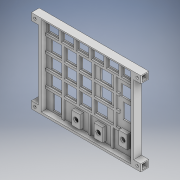
# Autodesk Inventor part: IPC Component Panel
Saved by Autodesk Inventor 2022 (Build 260153000, 153)
## iProperties
Created: 2021-12-31
Part Number: IPC Component Panel
Material: Generic
Document SubType Name: Modeling
Designer: solor
Density: 1 g/cm^3
Appearance: Default
Author: solor
Autodesk Inventor part; units mm, degrees
(part 1 of 2)
ref_plane "YZ Plane" through (0, 0, 0) normal (1, 0, 0) x (0, 1, 0)
ref_plane "XZ Plane" through (0, 0, 0) normal (0, 1, 0) x (-1, 0, 0)
ref_plane "XY Plane" through (0, 0, 0) normal (0, 0, 1) x (1, 0, 0)
sketch "Sketch1" plane through (0, 0, 0) normal (0, 0, 1) x (1, 0, 0)
  line L0 (-9, 0) -> (-9, -9)
  line L1 (-9, -46.5) -> (-9, -59.5)
  line L2 (-9, -97) -> (-9, -106)
  line L3 (-9, -9) -> (0, -9)
  line L4 (0, -9) -> (0, -46.5)
  line L5 (0, -46.5) -> (-9, -46.5)
  line L6 (-9, -59.5) -> (0, -59.5)
  line L7 (0, -59.5) -> (0, -97)
  line L8 (0, -97) -> (-9, -97)
  line L9 (-9, 0) -> (129.8502, 0)
  line L10 (129.8502, -9) -> (120.8502, -9)
  line L11 (120.8502, -9) -> (120.8502, -46.5)
  line L12 (120.8502, -46.5) -> (129.8502, -46.5)
  line L13 (129.8502, -46.5) -> (129.8502, -59.5)
  line L14 (129.8502, -59.5) -> (120.8502, -59.5)
  line L15 (120.8502, -59.5) -> (120.8502, -97)
  line L16 (120.8502, -97) -> (129.8502, -97)
  line L17 (129.8502, -97) -> (129.8502, -106)
  line L18 (-9, -106) -> (129.8502, -106)
  line L19 (129.8502, 0) -> (129.8502, -9)
  circle A0 centre (104.8902, -84.37) radius 6.22
  circle A1 centre (73.6502, -92.18) radius 3.05
  circle A2 centre (45.1902, -92.18) radius 3.05
  line L20 (21.7302, -100.81) -> (21.7302, -81.47)
  line L21 (21.7302, -81.47) -> (11.8502, -81.47)
  line L22 (11.8502, -81.47) -> (11.8502, -100.81)
  line L23 (11.8502, -100.81) -> (21.7302, -100.81)
  line L24 (100.7, -46.82) -> (110.58, -46.82)
  line L25 (110.58, -46.82) -> (110.58, -66.16)
  line L26 (110.58, -66.16) -> (100.7, -66.16)
  line L27 (100.7, -66.16) -> (100.7, -46.82)
  line L28 (5.7515, -17.0785) -> (19.8485, -17.0785)
  line L29 (19.8485, -17.0785) -> (19.8485, -2.9815)
  line L30 (19.8485, -2.9815) -> (5.7515, -2.9815)
  line L31 (5.7515, -2.9815) -> (5.7515, -17.0785)
  line L32 (5.7515, -17.0785) -> (19.8485, -2.9815) construction
  line L33 (19.8485, -17.0785) -> (5.7515, -2.9815) construction
  line L34 (24.8015, -17.0785) -> (38.8985, -17.0785)
  line L35 (38.8985, -17.0785) -> (38.8985, -2.9815)
  line L36 (38.8985, -2.9815) -> (24.8015, -2.9815)
  line L37 (24.8015, -2.9815) -> (24.8015, -17.0785)
  line L38 (24.8015, -17.0785) -> (38.8985, -2.9815) construction
  line L39 (38.8985, -17.0785) -> (24.8015, -2.9815) construction
  line L40 (43.8515, -17.0785) -> (57.9485, -17.0785)
  line L41 (57.9485, -17.0785) -> (57.9485, -2.9815)
  line L42 (57.9485, -2.9815) -> (43.8515, -2.9815)
  line L43 (43.8515, -2.9815) -> (43.8515, -17.0785)
  line L44 (43.8515, -17.0785) -> (57.9485, -2.9815) construction
  line L45 (57.9485, -17.0785) -> (43.8515, -2.9815) construction
  line L46 (62.9015, -17.0785) -> (76.9985, -17.0785)
  line L47 (76.9985, -17.0785) -> (76.9985, -2.9815)
  line L48 (76.9985, -2.9815) -> (62.9015, -2.9815)
  line L49 (62.9015, -2.9815) -> (62.9015, -17.0785)
  line L50 (62.9015, -17.0785) -> (76.9985, -2.9815) construction
  line L51 (76.9985, -17.0785) -> (62.9015, -2.9815) construction
  line L52 (81.9515, -17.0785) -> (96.0485, -17.0785)
  line L53 (96.0485, -17.0785) -> (96.0485, -2.9815)
  line L54 (96.0485, -2.9815) -> (81.9515, -2.9815)
  line L55 (81.9515, -2.9815) -> (81.9515, -17.0785)
  line L56 (81.9515, -17.0785) -> (96.0485, -2.9815) construction
  line L57 (96.0485, -17.0785) -> (81.9515, -2.9815) construction
  line L58 (101.0015, -17.0785) -> (115.0985, -17.0785)
  line L59 (115.0985, -17.0785) -> (115.0985, -2.9815)
  line L60 (115.0985, -2.9815) -> (101.0015, -2.9815)
  line L61 (101.0015, -2.9815) -> (101.0015, -17.0785)
  line L62 (101.0015, -17.0785) -> (115.0985, -2.9815) construction
  line L63 (115.0985, -17.0785) -> (101.0015, -2.9815) construction
  line L64 (9.4915, -37.4985) -> (23.5885, -37.4985)
  line L65 (23.5885, -37.4985) -> (23.5885, -23.4015)
  line L66 (23.5885, -23.4015) -> (9.4915, -23.4015)
  line L67 (9.4915, -23.4015) -> (9.4915, -37.4985)
  line L68 (9.4915, -37.4985) -> (23.5885, -23.4015) construction
  line L69 (23.5885, -37.4985) -> (9.4915, -23.4015) construction
  line L70 (28.5115, -37.4985) -> (42.6085, -37.4985)
  line L71 (42.6085, -37.4985) -> (42.6085, -23.4015)
  line L72 (42.6085, -23.4015) -> (28.5115, -23.4015)
  line L73 (28.5115, -23.4015) -> (28.5115, -37.4985)
  line L74 (28.5115, -37.4985) -> (42.6085, -23.4015) construction
  line L75 (42.6085, -37.4985) -> (28.5115, -23.4015) construction
  line L76 (47.5365, -37.4985) -> (61.6335, -37.4985)
  line L77 (61.6335, -37.4985) -> (61.6335, -23.4015)
  line L78 (61.6335, -23.4015) -> (47.5365, -23.4015)
  line L79 (47.5365, -23.4015) -> (47.5365, -37.4985)
  line L80 (47.5365, -37.4985) -> (61.6335, -23.4015) construction
  line L81 (61.6335, -37.4985) -> (47.5365, -23.4015) construction
  line L82 (72.1215, -37.4985) -> (86.2185, -37.4985)
  line L83 (86.2185, -37.4985) -> (86.2185, -23.4015)
  line L84 (86.2185, -23.4015) -> (72.1215, -23.4015)
  line L85 (72.1215, -23.4015) -> (72.1215, -37.4985)
  line L86 (72.1215, -37.4985) -> (86.2185, -23.4015) construction
  line L87 (86.2185, -37.4985) -> (72.1215, -23.4015) construction
  line L88 (98.5915, -41.7085) -> (112.6885, -41.7085)
  line L89 (112.6885, -41.7085) -> (112.6885, -27.6115)
  line L90 (112.6885, -27.6115) -> (98.5915, -27.6115)
  line L91 (98.5915, -27.6115) -> (98.5915, -41.7085)
  line L92 (98.5915, -41.7085) -> (112.6885, -27.6115) construction
  line L93 (112.6885, -41.7085) -> (98.5915, -27.6115) construction
  line L94 (9.4915, -56.5185) -> (23.5885, -56.5185)
  line L95 (23.5885, -56.5185) -> (23.5885, -42.4215)
  line L96 (23.5885, -42.4215) -> (9.4915, -42.4215)
  line L97 (9.4915, -42.4215) -> (9.4915, -56.5185)
  line L98 (9.4915, -56.5185) -> (23.5885, -42.4215) construction
  line L99 (23.5885, -56.5185) -> (9.4915, -42.4215) construction
  line L100 (28.5065, -56.5185) -> (42.6135, -56.5185)
  line L101 (42.6135, -56.5185) -> (42.6135, -42.4215)
  line L102 (42.6135, -42.4215) -> (28.5065, -42.4215)
  line L103 (28.5065, -42.4215) -> (28.5065, -56.5185)
  line L104 (28.5065, -56.5185) -> (42.6135, -42.4215) construction
  line L105 (42.6135, -56.5185) -> (28.5065, -42.4215) construction
  line L106 (47.5365, -56.5185) -> (61.6335, -56.5185)
  line L107 (61.6335, -56.5185) -> (61.6335, -42.4215)
  line L108 (61.6335, -42.4215) -> (47.5365, -42.4215)
  line L109 (47.5365, -42.4215) -> (47.5365, -56.5185)
  line L110 (47.5365, -56.5185) -> (61.6335, -42.4215) construction
  line L111 (61.6335, -56.5185) -> (47.5365, -42.4215) construction
  line L112 (72.1215, -56.5185) -> (86.2185, -56.5185)
  line L113 (86.2185, -56.5185) -> (86.2185, -42.4215)
  line L114 (86.2185, -42.4215) -> (72.1215, -42.4215)
  line L115 (72.1215, -42.4215) -> (72.1215, -56.5185)
  line L116 (72.1215, -56.5185) -> (86.2185, -42.4215) construction
  line L117 (86.2185, -56.5185) -> (72.1215, -42.4215) construction
  line L118 (9.5, -75.5385) -> (23.58, -75.5385)
  line L119 (23.58, -75.5385) -> (23.58, -61.4415)
  line L120 (23.58, -61.4415) -> (9.5, -61.4415)
  line L121 (9.5, -61.4415) -> (9.5, -75.5385)
  line L122 (9.5, -75.5385) -> (23.58, -61.4415) construction
  line L123 (23.58, -75.5385) -> (9.5, -61.4415) construction
  line L124 (28.5065, -75.5385) -> (42.6135, -75.5385)
  line L125 (42.6135, -75.5385) -> (42.6135, -61.4415)
  line L126 (42.6135, -61.4415) -> (28.5065, -61.4415)
  line L127 (28.5065, -61.4415) -> (28.5065, -75.5385)
  line L128 (28.5065, -75.5385) -> (42.6135, -61.4415) construction
  line L129 (42.6135, -75.5385) -> (28.5065, -61.4415) construction
  line L130 (47.5365, -75.5385) -> (61.6335, -75.5385)
  line L131 (61.6335, -75.5385) -> (61.6335, -61.4415)
  line L132 (61.6335, -61.4415) -> (47.5365, -61.4415)
  line L133 (47.5365, -61.4415) -> (47.5365, -75.5385)
  line L134 (47.5365, -75.5385) -> (61.6335, -61.4415) construction
  line L135 (61.6335, -75.5385) -> (47.5365, -61.4415) construction
  line L136 (66.6017, -75.5385) -> (80.6987, -75.5385)
  line L137 (80.6987, -75.5385) -> (80.6987, -61.4415)
  line L138 (80.6987, -61.4415) -> (66.6017, -61.4415)
  line L139 (66.6017, -61.4415) -> (66.6017, -75.5385)
  line L140 (66.6017, -75.5385) -> (80.6987, -61.4415) construction
  line L141 (80.6987, -75.5385) -> (66.6017, -61.4415) construction
  point P0 (0, 0)
  point P1 (0, 0)
  point P2 (12.8, -10.03)
  point P3 (31.85, -10.03)
  point P4 (50.9, -10.03)
  point P5 (69.95, -10.03)
  point P6 (89, -10.03)
  point P7 (10, -23.88)
  point P8 (16.54, -30.45)
  point P9 (35.56, -30.45)
  point P10 (54.585, -30.45)
  point P11 (79.17, -30.45)
  point P12 (79.17, -49.47)
  point P13 (54.585, -49.47)
  point P14 (35.56, -49.47)
  point P15 (16.54, -49.47)
  point P16 (16.54, -68.49)
  point P17 (35.56, -68.49)
  point P18 (54.585, -68.49)
  point P19 (73.6502, -68.49)
  point P20 (16.7902, -81.47)
  point P21 (21.7302, -91.14)
  point P22 (16.7902, -91.14)
  point P23 (110.58, -56.49)
  point P24 (105.64, -46.82)
  point P25 (105.64, -56.49)
  point P26 (108.05, -10.03)
  point P27 (105.64, -34.66)
  dimension "d56" = 14.097
  dimension "d57" = 14.097
  dimension "d58" = 14.097
  dimension "d59" = 14.097
  dimension "d60" = 14.097
  dimension "d61" = 14.097
  dimension "d62" = 14.097
  dimension "d63" = 14.097
  dimension "d65" = 14.097
  dimension "d66" = 14.097
  dimension "d67" = 14.097
  dimension "d68" = 14.097
  dimension "d69" = 14.097
  dimension "d72" = 14.097
  dimension "d73" = 14.097
  dimension "d74" = 14.097
  dimension "d75" = 14.097
  dimension "d76" = 14.097
  dimension "d77" = 14.097
  dimension "d78" = 14.107
  dimension "d79" = 14.097
  dimension "d80" = 14.097
  dimension "d81" = 14.097
  dimension "d82" = 14.097
  dimension "d83" = 14.097
  dimension "d84" = 14.097
  dimension "d85" = 14.097
  dimension "d86" = 14.097
  dimension "d87" = 14.097
  dimension "d88" = 14.097
  dimension "d89" = 14.107
  dimension "d90" = 14.097
  dimension "d91" = 14.08
  dimension "d92" = 19.34
  dimension "d144" = 6.1
  dimension "d145" = 6.1
  constraints: 284 end point, 42 midpoint, 38 parallel, 33 perpendicular, 27 point on line, 24 horizontal, 5 coincident, 4 vertical, 3 centre point
  measures "d56" distance of L30.end L29.end
  measures "d57" distance of L29.end L28.end
  measures "d58" distance of L36.end L35.end
  measures "d59" distance of L42.end L41.end
  measures "d60" distance of L48.end L47.end
  measures "d61" distance of L54.end L53.end
  measures "d62" distance of L60.end L59.end
  measures "d63" distance of L66.end L65.end
  measures "d65" distance of L72.end L71.end
  measures "d66" distance of L78.end L77.end
  measures "d67" distance of L84.end L83.end
  measures "d68" distance of L90.end L89.end
  measures "d69" distance of L89.end L88.end
  measures "d72" distance of L64.end L65.end
  measures "d73" distance of L70.end L71.end
  measures "d74" distance of L76.end L77.end
  measures "d75" distance of L82.end L83.end
  measures "d76" distance of L94.end L95.end
  measures "d77" distance of L95.end L96.end
  measures "d78" distance of L101.end L102.end
  measures "d79" distance of L100.end L101.end
  measures "d80" distance of L107.end L108.end
  measures "d81" distance of L106.end L107.end
  measures "d82" distance of L113.end L114.end
  measures "d83" distance of L112.end L113.end
  measures "d84" distance of L136.end L137.end
  measures "d85" distance of L137.end L138.end
  measures "d86" distance of L130.end L131.end
  measures "d87" distance of L131.end L132.end
  measures "d88" distance of L124.end L125.end
  measures "d89" distance of L125.end L126.end
  measures "d90" distance of L118.end L119.end
  measures "d91" distance of L119.end L120.end
  measures "d92" distance of L20.start L20.end
  measures "d144" diameter of A1
  measures "d145" diameter of A2
extrude "Extrusion1" add sketch "Sketch1" along normal blind 1.651
sketch "Sketch2" plane through (0, 0, 1.651) normal (0, 0, 1) x (1, 0, 0)
  line L0 (-9, 0) -> (-9, -9) projected
  line L1 (-9, -9) -> (0, -9) projected
  line L2 (0, -9) -> (0, -46.5) projected
  line L3 (0, -46.5) -> (-9, -46.5) projected
  line L4 (-9, -46.5) -> (-9, -59.5) projected
  line L5 (-9, -59.5) -> (0, -59.5) projected
  line L6 (0, -59.5) -> (0, -97) projected
  line L7 (0, -97) -> (-9, -97) projected
  line L8 (-9, -97) -> (-9, -106) projected
  line L9 (-9, -106) -> (129.8502, -106) projected
  line L10 (129.8502, -106) -> (129.8502, -97) projected
  line L11 (129.8502, -97) -> (120.8502, -97) projected
  line L12 (120.8502, -97) -> (120.8502, -59.5) projected
  line L13 (120.8502, -59.5) -> (129.8502, -59.5) projected
  line L14 (129.8502, -59.5) -> (129.8502, -46.5) projected
  line L15 (129.8502, -46.5) -> (120.8502, -46.5) projected
  line L16 (120.8502, -46.5) -> (120.8502, -9) projected
  line L17 (120.8502, -9) -> (129.8502, -9) projected
  line L18 (129.8502, -9) -> (129.8502, 0) projected
  line L19 (129.8502, 0) -> (-9, 0) projected
  circle A0 centre (104.8902, -84.37) radius 6.22 projected
  circle A1 centre (73.6502, -92.18) radius 3.05 projected
  circle A2 centre (45.1902, -92.18) radius 3.05 projected
  line L20 (66.6017, -75.5385) -> (66.6017, -61.4415) projected
  line L21 (66.6017, -61.4415) -> (80.6987, -61.4415) projected
  line L22 (80.6987, -61.4415) -> (80.6987, -75.5385) projected
  line L23 (80.6987, -75.5385) -> (66.6017, -75.5385) projected
  line L24 (47.5365, -75.5385) -> (47.5365, -61.4415) projected
  line L25 (47.5365, -61.4415) -> (61.6335, -61.4415) projected
  line L26 (61.6335, -61.4415) -> (61.6335, -75.5385) projected
  line L27 (61.6335, -75.5385) -> (47.5365, -75.5385) projected
  line L28 (28.5065, -75.5385) -> (28.5065, -61.4415) projected
  line L29 (28.5065, -61.4415) -> (42.6135, -61.4415) projected
  line L30 (42.6135, -61.4415) -> (42.6135, -75.5385) projected
  line L31 (42.6135, -75.5385) -> (28.5065, -75.5385) projected
  line L32 (9.5, -75.5385) -> (9.5, -61.4415) projected
  line L33 (9.5, -61.4415) -> (23.58, -61.4415) projected
  line L34 (23.58, -61.4415) -> (23.58, -75.5385) projected
  line L35 (23.58, -75.5385) -> (9.5, -75.5385) projected
  line L36 (72.1215, -56.5185) -> (72.1215, -42.4215) projected
  line L37 (72.1215, -42.4215) -> (86.2185, -42.4215) projected
  line L38 (86.2185, -42.4215) -> (86.2185, -56.5185) projected
  line L39 (86.2185, -56.5185) -> (72.1215, -56.5185) projected
  line L40 (47.5365, -56.5185) -> (47.5365, -42.4215) projected
  line L41 (47.5365, -42.4215) -> (61.6335, -42.4215) projected
  line L42 (61.6335, -42.4215) -> (61.6335, -56.5185) projected
  line L43 (61.6335, -56.5185) -> (47.5365, -56.5185) projected
  line L44 (28.5065, -56.5185) -> (28.5065, -42.4215) projected
  line L45 (28.5065, -42.4215) -> (42.6135, -42.4215) projected
  line L46 (42.6135, -42.4215) -> (42.6135, -56.5185) projected
  line L47 (42.6135, -56.5185) -> (28.5065, -56.5185) projected
  line L48 (9.4915, -56.5185) -> (9.4915, -42.4215) projected
  line L49 (9.4915, -42.4215) -> (23.5885, -42.4215) projected
  line L50 (23.5885, -42.4215) -> (23.5885, -56.5185) projected
  line L51 (23.5885, -56.5185) -> (9.4915, -56.5185) projected
  line L52 (98.5915, -41.7085) -> (98.5915, -27.6115) projected
  line L53 (98.5915, -27.6115) -> (112.6885, -27.6115) projected
  line L54 (112.6885, -27.6115) -> (112.6885, -41.7085) projected
  line L55 (112.6885, -41.7085) -> (98.5915, -41.7085) projected
  line L56 (72.1215, -37.4985) -> (72.1215, -23.4015) projected
  line L57 (72.1215, -23.4015) -> (86.2185, -23.4015) projected
  line L58 (86.2185, -23.4015) -> (86.2185, -37.4985) projected
  line L59 (86.2185, -37.4985) -> (72.1215, -37.4985) projected
  line L60 (47.5365, -37.4985) -> (47.5365, -23.4015) projected
  line L61 (47.5365, -23.4015) -> (61.6335, -23.4015) projected
  line L62 (61.6335, -23.4015) -> (61.6335, -37.4985) projected
  line L63 (61.6335, -37.4985) -> (47.5365, -37.4985) projected
  line L64 (28.5115, -37.4985) -> (28.5115, -23.4015) projected
  line L65 (28.5115, -23.4015) -> (42.6085, -23.4015) projected
  line L66 (42.6085, -23.4015) -> (42.6085, -37.4985) projected
  line L67 (42.6085, -37.4985) -> (28.5115, -37.4985) projected
  line L68 (9.4915, -37.4985) -> (9.4915, -23.4015) projected
  line L69 (9.4915, -23.4015) -> (23.5885, -23.4015) projected
  line L70 (23.5885, -23.4015) -> (23.5885, -37.4985) projected
  line L71 (23.5885, -37.4985) -> (9.4915, -37.4985) projected
  line L72 (101.0015, -17.0785) -> (101.0015, -2.9815) projected
  line L73 (101.0015, -2.9815) -> (115.0985, -2.9815) projected
  line L74 (115.0985, -2.9815) -> (115.0985, -17.0785) projected
  line L75 (115.0985, -17.0785) -> (101.0015, -17.0785) projected
  line L76 (81.9515, -17.0785) -> (81.9515, -2.9815) projected
  line L77 (81.9515, -2.9815) -> (96.0485, -2.9815) projected
  line L78 (96.0485, -2.9815) -> (96.0485, -17.0785) projected
  line L79 (96.0485, -17.0785) -> (81.9515, -17.0785) projected
  line L80 (62.9015, -17.0785) -> (62.9015, -2.9815) projected
  line L81 (62.9015, -2.9815) -> (76.9985, -2.9815) projected
  line L82 (76.9985, -2.9815) -> (76.9985, -17.0785) projected
  line L83 (76.9985, -17.0785) -> (62.9015, -17.0785) projected
  line L84 (43.8515, -17.0785) -> (43.8515, -2.9815) projected
  line L85 (43.8515, -2.9815) -> (57.9485, -2.9815) projected
  line L86 (57.9485, -2.9815) -> (57.9485, -17.0785) projected
  line L87 (57.9485, -17.0785) -> (43.8515, -17.0785) projected
  line L88 (24.8015, -17.0785) -> (24.8015, -2.9815) projected
  line L89 (24.8015, -2.9815) -> (38.8985, -2.9815) projected
  line L90 (38.8985, -2.9815) -> (38.8985, -17.0785) projected
  line L91 (38.8985, -17.0785) -> (24.8015, -17.0785) projected
  line L92 (5.7515, -17.0785) -> (5.7515, -2.9815) projected
  line L93 (5.7515, -2.9815) -> (19.8485, -2.9815) projected
  line L94 (19.8485, -2.9815) -> (19.8485, -17.0785) projected
  line L95 (19.8485, -17.0785) -> (5.7515, -17.0785) projected
  line L96 (100.7, -46.82) -> (110.58, -46.82) projected
  line L97 (110.58, -46.82) -> (110.58, -66.16) projected
  line L98 (110.58, -66.16) -> (100.7, -66.16) projected
  line L99 (100.7, -66.16) -> (100.7, -46.82) projected
  line L100 (21.7302, -100.81) -> (11.8502, -100.81) projected
  line L101 (11.8502, -100.81) -> (11.8502, -81.47) projected
  line L102 (11.8502, -81.47) -> (21.7302, -81.47) projected
  line L103 (21.7302, -81.47) -> (21.7302, -100.81) projected
  line L104 (19.8485, -2.9815) -> (19.8485, -17.0785) construction
  line L105 (24.8015, -17.0785) -> (24.8015, -2.9815) construction
  line L106 (19.8485, -17.0785) -> (5.7515, -17.0785) construction
  line L107 (61.6335, -23.4015) -> (61.6335, -37.4985) construction
  line L108 (61.6335, -26.759) -> (72.1215, -26.759) construction
  line L109 (72.1215, -37.4985) -> (72.1215, -23.4015) construction
  line L110 (61.6335, -37.4985) -> (47.5365, -37.4985) construction
  line L111 (47.5365, -42.4215) -> (61.6335, -42.4215) construction
  line L112 (9.5, -61.4415) -> (23.58, -61.4415) construction
  line L113 (61.6335, -61.4415) -> (61.6335, -75.5385) construction
  line L114 (61.6335, -68.49) -> (66.6017, -68.49) construction
  line L115 (97.4975, -57.48) -> (97.4975, -60.48)
  line L116 (9.5, -57.48) -> (9.5, -60.48)
  line L117 (97.4975, -38.46) -> (97.4975, -41.46)
  line L118 (9.5, -38.46) -> (9.5, -41.46)
  line L119 (97.4975, -57.48) -> (97.4975, -60.48)
  line L120 (9.5, -57.48) -> (9.5, -60.48)
  line L121 (97.4975, -38.46) -> (97.4975, -41.46)
  line L122 (9.5, -38.46) -> (9.5, -41.46)
  line L123 (97.4975, -76.75) -> (97.4975, -79.75)
  line L124 (9.5, -76.75) -> (9.5, -79.75)
  line L125 (9.5, -38.46) -> (9.5, -41.46)
  line L126 (9.5, -38.46) -> (9.5, -41.46)
  line L127 (7.0425, -18.74) -> (7.0425, -21.74)
  line L128 (7.0425, -18.74) -> (7.0425, -21.74)
  line L129 (113.8947, -18.74) -> (113.8947, -21.74)
  line L130 (22.325, -2.9815) -> (23.825, -2.9815)
  line L131 (23.825, -2.9815) -> (23.825, -18.74)
  line L132 (22.325, -2.9815) -> (20.825, -2.9815)
  line L133 (20.825, -2.9815) -> (20.825, -18.74)
  line L134 (7.0425, -18.74) -> (20.825, -18.74)
  line L135 (23.5885, -23.4015) -> (23.5885, -37.4985) projected
  line L136 (27.55, -21.74) -> (27.55, -38.46)
  line L137 (24.55, -21.74) -> (24.55, -38.46)
  line L138 (9.5, -38.46) -> (24.55, -38.46)
  line L139 (24.55, -21.74) -> (7.0425, -21.74)
  line L140 (9.5, -38.46) -> (24.55, -38.46)
  line L141 (24.55, -100.81) -> (27.55, -100.81)
  line L142 (9.5, -41.46) -> (24.55, -41.46)
  line L143 (9.5, -57.48) -> (24.55, -57.48)
  line L144 (9.5, -57.48) -> (24.55, -57.48)
  line L145 (9.5, -60.48) -> (24.55, -60.48)
  line L146 (24.55, -41.46) -> (24.55, -57.48)
  line L147 (27.55, -57.48) -> (27.55, -41.46)
  line L148 (9.5, -60.48) -> (24.55, -60.48)
  line L149 (9.5, -41.46) -> (24.55, -41.46)
  line L150 (9.5, -76.75) -> (24.55, -76.75)
  line L151 (27.55, -100.81) -> (27.55, -79.75)
  line L152 (27.55, -76.75) -> (27.55, -60.48)
  line L153 (9.5, -79.75) -> (24.55, -79.75)
  line L154 (24.55, -60.48) -> (24.55, -76.75)
  line L155 (24.55, -79.75) -> (24.55, -100.81)
  line L156 (43.8515, -2.9815) -> (57.9485, -2.9815) projected
  line L157 (39.875, -2.9815) -> (39.875, -18.74)
  line L158 (42.875, -18.74) -> (42.875, -2.9815)
  line L159 (23.825, -18.74) -> (39.875, -18.74)
  line L160 (57.9485, -2.9815) -> (57.9485, -17.0785) projected
  line L161 (39.875, -2.9815) -> (42.875, -2.9815)
  line L162 (39.875, -2.9815) -> (39.875, -18.74)
  line L163 (42.875, -18.74) -> (42.875, -2.9815)
  line L164 (39.875, -2.9815) -> (42.875, -2.9815)
  line L165 (58.925, -2.9815) -> (58.925, -18.74)
  line L166 (61.925, -18.74) -> (61.925, -2.9815)
  line L167 (58.925, -2.9815) -> (61.925, -2.9815)
  line L168 (77.975, -2.9815) -> (77.975, -18.74)
  line L169 (80.975, -18.74) -> (80.975, -2.9815)
  line L170 (77.975, -2.9815) -> (80.975, -2.9815)
  line L171 (97.025, -2.9815) -> (97.025, -18.74)
  line L172 (100.025, -18.74) -> (100.025, -2.9815)
  line L173 (97.025, -2.9815) -> (100.025, -2.9815)
  line L174 (42.875, -18.74) -> (58.925, -18.74)
  line L175 (61.925, -18.74) -> (77.975, -18.74)
  line L176 (80.975, -18.74) -> (97.025, -18.74)
  line L177 (100.025, -18.74) -> (113.8947, -18.74)
  line L178 (42.6085, -23.4015) -> (42.6085, -37.4985) projected
  line L179 (47.5365, -37.4985) -> (47.5365, -23.4015) projected
  line L180 (27.55, -38.46) -> (43.5725, -38.46)
  line L181 (27.55, -38.46) -> (43.5725, -38.46)
  line L182 (43.5725, -38.46) -> (43.5725, -21.74)
  line L183 (43.5725, -38.46) -> (43.5725, -21.74)
  line L184 (27.55, -41.46) -> (43.5725, -41.46)
  line L185 (27.55, -41.46) -> (43.5725, -41.46)
  line L186 (46.5725, -21.74) -> (46.5725, -38.46)
  line L187 (46.5725, -21.74) -> (46.5725, -38.46)
  line L188 (43.5725, -21.74) -> (27.55, -21.74)
  line L189 (62.5975, -21.74) -> (46.5725, -21.74)
  line L190 (46.5725, -38.46) -> (62.5975, -38.46)
  line L191 (46.5725, -38.46) -> (62.5975, -38.46)
  line L192 (62.5975, -38.46) -> (62.5975, -21.74)
  line L193 (46.5725, -41.46) -> (62.5975, -41.46)
  line L194 (46.5725, -41.46) -> (62.5975, -41.46)
  line L195 (65.5975, -21.74) -> (65.5975, -38.46)
  line L196 (62.5975, -76.75) -> (62.5975, -60.48)
  line L197 (62.5975, -57.48) -> (62.5975, -41.46)
  line L198 (65.5975, -41.46) -> (65.5975, -57.48)
  line L199 (65.5975, -60.48) -> (65.5975, -76.75)
  line L200 (27.55, -60.48) -> (43.5725, -60.48)
  line L201 (46.5725, -60.48) -> (62.5975, -60.48)
  line L202 (27.55, -60.48) -> (43.5725, -60.48)
  line L203 (46.5725, -60.48) -> (62.5975, -60.48)
  line L204 (43.5725, -76.75) -> (43.5725, -60.48)
  line L205 (43.5725, -57.48) -> (43.5725, -41.46)
  line L206 (43.5725, -76.75) -> (43.5725, -60.48)
  line L207 (43.5725, -57.48) -> (43.5725, -41.46)
  line L208 (27.55, -57.48) -> (43.5725, -57.48)
  line L209 (46.5725, -57.48) -> (62.5975, -57.48)
  line L210 (27.55, -57.48) -> (43.5725, -57.48)
  line L211 (46.5725, -57.48) -> (62.5975, -57.48)
  line L212 (46.5725, -41.46) -> (46.5725, -57.48)
  line L213 (46.5725, -60.48) -> (46.5725, -76.75)
  line L214 (46.5725, -41.46) -> (46.5725, -57.48)
  line L215 (46.5725, -60.48) -> (46.5725, -76.75)
  line L216 (27.55, -76.75) -> (43.5725, -76.75)
  line L217 (46.5725, -76.75) -> (62.5975, -76.75)
  line L218 (65.5975, -76.75) -> (90.6137, -76.75)
  line L219 (93.6137, -76.75) -> (97.4975, -76.75)
  line L220 (65.5975, -60.48) -> (90.6137, -60.48)
  line L221 (93.6137, -60.48) -> (97.4975, -60.48)
  line L222 (65.5975, -60.48) -> (90.6137, -60.48)
  line L223 (93.6137, -60.48) -> (97.4975, -60.48)
  line L224 (93.6137, -60.48) -> (93.6137, -76.75)
  line L225 (90.6137, -76.75) -> (90.6137, -60.48)
  line L226 (65.5975, -57.48) -> (90.6137, -57.48)
  line L227 (93.6137, -57.48) -> (97.4975, -57.48)
  line L228 (65.5975, -57.48) -> (90.6137, -57.48)
  line L229 (93.6137, -57.48) -> (97.4975, -57.48)
  line L230 (65.5975, -41.46) -> (90.6137, -41.46)
  line L231 (93.6137, -41.46) -> (97.4975, -41.46)
  line L232 (65.5975, -41.46) -> (90.6137, -41.46)
  line L233 (93.6137, -41.46) -> (97.4975, -41.46)
  line L234 (93.6137, -21.74) -> (93.6137, -38.46)
  line L235 (93.6137, -41.46) -> (93.6137, -57.48)
  line L236 (65.5975, -38.46) -> (90.6137, -38.46)
  line L237 (93.6137, -38.46) -> (97.4975, -38.46)
  line L238 (65.5975, -38.46) -> (90.6137, -38.46)
  line L239 (93.6137, -38.46) -> (97.4975, -38.46)
  line L240 (90.6137, -57.48) -> (90.6137, -41.46)
  line L241 (90.6137, -38.46) -> (90.6137, -21.74)
  line L242 (57.9485, -79.75) -> (57.9485, -100.81)
  line L243 (57.9485, -100.81) -> (60.9485, -100.81)
  line L244 (60.9485, -100.81) -> (60.9485, -79.75)
  line L245 (86.7283, -79.75) -> (86.7283, -100.81)
  line L246 (86.7283, -100.81) -> (89.7283, -100.81)
  line L247 (89.7283, -100.81) -> (89.7283, -79.75)
  line L248 (27.55, -79.75) -> (57.9485, -79.75)
  line L249 (60.9485, -79.75) -> (86.7283, -79.75)
  line L250 (89.7283, -79.75) -> (97.4975, -79.75)
  line L251 (113.8947, -21.74) -> (93.6137, -21.74)
  line L252 (90.6137, -21.74) -> (65.5975, -21.74)
  point P0 (0, 0)
  point P1 (14.3078, -58.98)
  point P2 (14.3078, -39.96)
  point P3 (14.3078, -39.96)
  point P4 (14.3078, -58.98)
  point P5 (14.3078, -39.96)
  point P6 (14.3078, -39.96)
  point P7 (14.3078, -78.25)
  point P8 (14.3078, -78.25)
  point P9 (11.8502, -20.24)
  point P10 (11.8502, -20.24)
  dimension "d102" = 1.5
  dimension "d103" = 1.5
  dimension "d114" = 3
  dimension "d115" = 3
  constraints: 270 end point, 151 perpendicular, 33 horizontal, 10 vertical, 4 point on line, 2 coincident, 2 midpoint, 1 collinear, 1 parallel
  measures "d102" distance of L130.start L130.end
  measures "d103" distance of L130.start L132.end
  measures "d114" distance of L242.end L243.end
  measures "d115" distance of L245.end L246.end
extrude "Extrusion2" add sketch "Sketch2" along normal blind 2 contours L115 L221 L224 L219 L123 L250 L247 L246 L245 L249 L244 L243 L242 L248 L151 L141 L155 L153 L124 L150 L154 L145 L116 L143 L146 L142 L118 L138 L137 L139 L127 L134 L133 L132 L130 L131 L159 L157 L161 L158 L174 L165 L167 L166 L175 L168 L170 L169 L176 L171 L173 L172 L177 L129 L251 L234 L237 L117 L231 L235 L227
sketch "Sketch3" plane through (0, 0, 1.651) normal (0, 0, 1) x (1, 0, 0)
  line L0 (0, -59.5) -> (0, -97) projected
  line L1 (0, -59.5) -> (0, -97) projected
  line L2 (0, -63.897) -> (0, -41.177)
  line L3 (0, -9) -> (0, -46.5) projected
  line L4 (0, -41.177) -> (-17.7441, -43.618)
  line L5 (-17.7441, -43.618) -> (-15.4103, -60.5836)
  line L6 (-15.4103, -60.5836) -> (0, -63.897)
  line L7 (120.8502, -97) -> (120.8502, -59.5) projected
  line L8 (120.8502, -63.897) -> (120.8502, -38.9238)
  line L9 (120.8502, -38.9238) -> (132.4709, -38.9238)
  line L10 (132.4709, -38.9238) -> (132.4709, -63.897)
  line L11 (132.4709, -63.897) -> (120.8502, -63.897)
  point P0 (0, 0)
  constraints: 16 end point, 4 perpendicular, 3 point on line, 1 collinear
extrude "Extrusion3" cut sketch "Sketch3" against normal blind 2
sketch "Sketch4" plane through (0, 0, 1.651) normal (0, 0, 1) x (1, 0, 0)
  line L0 (0, 0) -> (0, -106)
  line L1 (-9, -106) -> (129.8502, -106) projected
  line L2 (120.8502, -97) -> (120.8502, -9) projected
  line L3 (0, -106) -> (120.8502, -106)
  line L4 (120.8502, -106) -> (120.8502, 0)
  line L5 (129.8502, 0) -> (-9, 0) projected
  line L6 (120.8502, 0) -> (0, 0)
  line L7 (1.5596, -1.5596) -> (119.2906, -1.5596)
  line L8 (3.5261, -1.5596) -> (3.5261, -103.1629)
  line L9 (3.5261, -103.1629) -> (117.3241, -103.1629)
  line L10 (117.3241, -103.1629) -> (117.3241, -1.5596)
  point P0 (120.8502, -9)
  dimension "d120" = 113.798
  constraints: 16 end point, 5 point on line, 4 perpendicular, 1 parallel, 1 vertical
  measures "d120" distance of L8.end L9.end
extrude "Extrusion4" add sketch "Sketch4" along normal blind 12
sketch "Sketch5" plane through (0, 0, 1.651) normal (0, 0, 1) x (1, 0, 0)
  line L0 (0, -9) -> (0, -97) projected
  line L1 (-9, -9) -> (0, -9) projected
  line L2 (0, -9) -> (-9, -9)
  line L3 (129.8502, 0) -> (-9, 0) projected
  line L4 (-9, -9) -> (-9, 0)
  line L5 (-9, 0) -> (0, 0)
  line L6 (120.8502, 0) -> (0, 0) projected
  line L7 (0, -9) -> (0, 0)
  line L8 (120.8502, 0) -> (129.8502, 0)
  line L9 (129.8502, -9) -> (129.8502, 0) projected
  line L10 (129.8502, 0) -> (129.8502, -9)
  line L11 (120.8502, -97) -> (120.8502, -9) projected
  line L12 (129.8502, -9) -> (120.8502, -9)
  line L13 (120.8502, -9) -> (120.8502, 0)
  line L14 (-9, -106) -> (129.8502, -106) projected
  line L15 (129.8502, -97) -> (129.8502, -106)
  line L16 (129.8502, -106) -> (120.8502, -106)
  line L17 (0, -106) -> (120.8502, -106) projected
  line L18 (120.8502, -106) -> (120.8502, -97)
  line L19 (129.8502, -97) -> (120.8502, -97) projected
  line L20 (120.8502, -97) -> (129.8502, -97)
  line L21 (0, -97) -> (-9, -97) projected
  line L22 (-9, -97) -> (0, -97)
  line L23 (0, -97) -> (0, -106)
  line L24 (0, -106) -> (-9, -106)
  line L25 (-9, -97) -> (-9, -106) projected
  line L26 (-9, -106) -> (-9, -97)
  constraints: 32 end point, 7 collinear, 4 perpendicular, 2 point on line, 2 vertical, 1 horizontal
extrude "Extrusion5" add sketch "Sketch5" along normal blind 1.016 contours L1 L4 L3 L7 | L23 L14 L25 L21 | L3 L9 L12 L13 | L18 L19 L15 L14
sketch "Sketch6" plane through (0, 0, 2.667) normal (0, 0, 1) x (1, 0, 0)
  line L0 (-9, -9) -> (0, -9) projected
  line L1 (-9, 0) -> (-9, -9) projected
  line L2 (-9, -97) -> (-9, -106) projected
  line L3 (129.8502, -97) -> (120.8502, -97) projected
  circle A0 centre (-4.5, -4.5) radius 1.65
  circle A1 centre (125.3502, -4.5) radius 1.65
  circle A2 centre (125.3502, -101.5) radius 1.65
  circle A3 centre (-4.5, -101.5) radius 1.65
  point P0 (0, 0)
  point P1 (-4.5, -9)
  point P2 (-9, -4.5)
  point P3 (-9, -101.5)
  point P4 (125.3502, -97)
  dimension "d125" = 3.3
  constraints: 4 centre point, 4 coincident, 4 midpoint
  measures "d125" diameter of A0
extrude "Extrusion6" cut sketch "Sketch6" against normal blind 10.541
sketch "Sketch7" plane through (0, 0, 3.651) normal (0, 0, 1) x (1, 0, 0)
  line L0 (7.0425, -18.74) -> (20.825, -18.74) projected
  line L1 (7.0425, -18.74) -> (3.5261, -18.74)
  line L2 (3.5261, -1.5596) -> (3.5261, -103.1629) projected
  line L3 (7.0425, -18.74) -> (7.0425, -21.74) projected
  line L4 (7.0425, -21.74) -> (3.5261, -21.74)
  line L5 (3.5261, -21.74) -> (3.5261, -18.74)
  line L6 (9.5, -38.46) -> (24.55, -38.46) projected
  line L7 (9.5, -38.46) -> (3.5261, -38.46)
  line L8 (3.5261, -38.46) -> (3.5261, -41.46)
  line L9 (9.5, -41.46) -> (24.55, -41.46) projected
  line L10 (3.5261, -41.46) -> (9.5, -41.46)
  line L11 (9.5, -41.46) -> (9.5, -38.46)
  line L12 (24.55, -57.48) -> (9.5, -57.48) projected
  line L13 (9.5, -57.48) -> (3.5261, -57.48)
  line L14 (9.5, -60.48) -> (24.55, -60.48) projected
  line L15 (9.5, -57.48) -> (9.5, -60.48)
  line L16 (9.5, -60.48) -> (3.5261, -60.48)
  line L17 (3.5261, -60.48) -> (3.5261, -57.48)
  line L18 (9.5, -79.75) -> (24.55, -79.75) projected
  line L19 (9.5, -79.75) -> (3.5261, -79.75)
  line L20 (9.5, -76.75) -> (9.5, -79.75) projected
  line L21 (9.5, -79.75) -> (9.5, -76.75)
  line L22 (9.5, -76.75) -> (3.5261, -76.75)
  line L23 (3.5261, -76.75) -> (3.5261, -79.75)
  line L24 (24.55, -100.81) -> (27.55, -100.81) projected
  line L25 (24.55, -100.81) -> (24.55, -103.1629)
  line L26 (3.5261, -103.1629) -> (117.3241, -103.1629) projected
  line L27 (24.55, -100.81) -> (27.55, -100.81)
  line L28 (27.55, -100.81) -> (27.55, -103.1629)
  line L29 (27.55, -103.1629) -> (24.55, -103.1629)
  line L30 (57.9485, -100.81) -> (60.9485, -100.81) projected
  line L31 (57.9485, -100.81) -> (60.9485, -100.81)
  line L32 (60.9485, -100.81) -> (60.9485, -103.1629)
  line L33 (60.9485, -103.1629) -> (57.9485, -103.1629)
  line L34 (57.9485, -79.75) -> (57.9485, -100.81) projected
  line L35 (57.9485, -100.81) -> (57.9485, -103.1629)
  line L36 (89.7283, -100.81) -> (86.7283, -100.81) projected
  line L37 (86.7283, -100.81) -> (89.7283, -100.81)
  line L38 (89.7283, -100.81) -> (89.7283, -103.1629)
  line L39 (89.7283, -103.1629) -> (86.7283, -103.1629)
  line L40 (86.7283, -103.1629) -> (86.7283, -100.81)
  line L41 (113.8947, -21.74) -> (113.8947, -18.74) projected
  line L42 (113.8947, -18.74) -> (113.8947, -21.74)
  line L43 (113.8947, -21.74) -> (117.3241, -21.74)
  line L44 (117.3241, -103.1629) -> (117.3241, -1.5596) projected
  line L45 (117.3241, -21.74) -> (117.3241, -18.74)
  line L46 (117.3241, -18.74) -> (113.8947, -18.74)
  line L47 (100.025, -18.74) -> (100.025, -2.9815) projected
  line L48 (100.025, -2.9815) -> (100.025, -1.5596)
  line L49 (117.3241, -1.5596) -> (3.5261, -1.5596) projected
  line L50 (100.025, -2.9815) -> (97.025, -2.9815) projected
  line L51 (100.025, -2.9815) -> (97.025, -2.9815)
  line L52 (97.025, -2.9815) -> (97.025, -1.5596)
  line L53 (97.025, -1.5596) -> (100.025, -1.5596)
  line L54 (80.975, -2.9815) -> (77.975, -2.9815) projected
  line L55 (80.975, -2.9815) -> (77.975, -2.9815)
  line L56 (77.975, -2.9815) -> (77.975, -1.5596)
  line L57 (77.975, -1.5596) -> (80.975, -1.5596)
  line L58 (80.975, -18.74) -> (80.975, -2.9815) projected
  line L59 (80.975, -1.5596) -> (80.975, -2.9815)
  line L60 (61.925, -2.9815) -> (58.925, -2.9815) projected
  line L61 (58.925, -2.9815) -> (61.925, -2.9815)
  line L62 (61.925, -2.9815) -> (61.925, -1.5596)
  line L63 (61.925, -1.5596) -> (58.925, -1.5596)
  line L64 (58.925, -1.5596) -> (58.925, -2.9815)
  line L65 (42.875, -18.74) -> (42.875, -2.9815) projected
  line L66 (42.875, -2.9815) -> (39.875, -2.9815) projected
  line L67 (42.875, -2.9815) -> (39.875, -2.9815)
  line L68 (39.875, -2.9815) -> (39.875, -1.5596)
  line L69 (39.875, -1.5596) -> (42.875, -1.5596)
  line L70 (42.875, -1.5596) -> (42.875, -2.9815)
  line L71 (23.825, -18.74) -> (23.825, -2.9815) projected
  line L72 (23.825, -2.9815) -> (20.825, -2.9815) projected
  line L73 (23.825, -2.9815) -> (20.825, -2.9815)
  line L74 (20.825, -2.9815) -> (20.825, -1.5596)
  line L75 (20.825, -1.5596) -> (23.825, -1.5596)
  line L76 (23.825, -1.5596) -> (23.825, -2.9815)
  point P0 (0, 0)
  constraints: 102 end point, 25 perpendicular, 17 point on line, 9 collinear, 4 horizontal, 4 vertical, 1 parallel, 8 other
extrude "Extrusion7" add sketch "Sketch7" against normal blind 2 contours L3 L4 L2 L1 | L49 L76 L72 L74 | L7 L11 L10 L2 | L49 L70 L66 L68 | L13 L15 L16 L2 | L49 L62 L60 L64 | L22 L20 L19 L2 | L49 L59 L54 L56 | L25 L24 L28 L26 | L49 L48 L50 L52 | L35 L30 L32 L26 | L44 L43 L41 L46 | L40 L36 L38 L26
sketch "Sketch8" plane through (0, 0, 13.651) normal (0, 0, 1) x (1, 0, 0)
  circle A0 centre (-4.5, -4.5) radius 1.65 projected
  line L0 (-9, -9) -> (0, -9) projected
  line L1 (0, 0) -> (0, -9) projected
  line L2 (0, 0) -> (-9, 0) projected
  line L3 (-9, 0) -> (-9, -9) projected
  circle A1 centre (125.3502, -4.5) radius 1.65 projected
  line L4 (129.8502, -9) -> (129.8502, 0) projected
  line L5 (129.8502, 0) -> (120.8502, 0) projected
  line L6 (120.8502, -9) -> (120.8502, 0) projected
  line L7 (120.8502, -9) -> (129.8502, -9) projected
  circle A2 centre (125.3502, -101.5) radius 1.65 projected
  line L8 (129.8502, -97) -> (120.8502, -97) projected
  line L9 (120.8502, -106) -> (120.8502, -97) projected
  line L10 (120.8502, -106) -> (129.8502, -106) projected
  line L11 (129.8502, -106) -> (129.8502, -97) projected
  circle A3 centre (-4.5, -101.5) radius 1.65 projected
  circle A4 centre (-4.5, -101.5) radius 1.65 projected
  line L12 (-9, -106) -> (0, -106) projected
  line L13 (0, -97) -> (0, -106) projected
  line L14 (0, -97) -> (-9, -97) projected
  line L15 (-9, -97) -> (-9, -106) projected
extrude "Extrusion8" add sketch "Sketch8" against normal blind 2.62
sketch "Sketch9" plane through (-9, -106, 0) normal (0, -1, 0) x (1, 0, 0)
  line L0 (129.8502, 11.031) -> (138.8502, 11.031) projected
  line L1 (138.8502, 2.667) -> (129.8502, 2.667) projected
  line L2 (138.8502, 11.031) -> (138.8502, 2.667)
  line L3 (138.8502, 2.667) -> (129.8502, 2.667)
  line L4 (129.8502, 2.667) -> (129.8502, 11.031) projected
  line L5 (129.8502, 2.667) -> (129.8502, 11.031)
  line L6 (138.8502, 13.651) -> (138.8502, 11.031) projected
  line L7 (129.8502, 11.031) -> (138.8502, 11.031)
  line L8 (9, 2.667) -> (0, 2.667) projected
  line L9 (0, 13.651) -> (0, 11.031) projected
  line L10 (0, 2.667) -> (0, 11.031)
  line L11 (9, 2.667) -> (9, 11.031) projected
  line L12 (0, 11.031) -> (9, 11.031)
  line L13 (9, 11.031) -> (9, 2.667)
  line L14 (0, 0) -> (0, 2.667) projected
  line L15 (9, 2.667) -> (0, 2.667)
  point P0 (9, 0)
  constraints: 16 end point, 5 perpendicular, 2 vertical, 1 collinear
extrude "Extrusion9" add sketch "Sketch9" against normal blind 113.2675
sketch "Sketch10" plane through (129.8502, -106, 0) normal (1, 0, 0) x (0, 0, -1)
  line L0 (-13.651, 9) -> (-11.031, 9) projected
  line L1 (0, 9) -> (-2.667, 9) projected
  line L2 (-11.031, 9) -> (-2.667, 9)
  line L3 (0, 97) -> (-2.667, 97) projected
  line L4 (-2.667, 9) -> (-2.667, 97)
  line L5 (-2.667, 97) -> (-11.031, 97)
  line L6 (-11.031, 97) -> (-11.031, 9) projected
  line L7 (-11.031, 97) -> (-11.031, 9)
  line L8 (-13.651, 2.85) -> (-13.651, 6.15) projected
  line L9 (-13.651, 99.85) -> (-13.651, 103.15) projected
  line L10 (-11.031, 9) -> (-11.031, 7.7)
  line L11 (-11.031, 6.15) -> (-13.651, 6.15) projected
  line L12 (-11.031, 7.7) -> (-2.667, 7.7)
  line L13 (-3.651, 26.25) -> (-3.651, 2.8371) projected
  line L14 (-2.667, 7.7) -> (-2.667, 1.3)
  line L15 (0, 0) -> (-13.651, 0) projected
  line L16 (-2.667, 1.3) -> (-11.031, 1.3)
  line L17 (-11.031, 1.3) -> (-11.031, 7.7)
  line L18 (-2.667, 97) -> (-2.667, 98.3)
  line L19 (-2.667, 98.3) -> (-11.031, 98.3)
  line L20 (-11.031, 98.3) -> (-11.031, 104.7)
  line L21 (-11.031, 104.7) -> (-2.667, 104.7)
  line L22 (-2.667, 104.7) -> (-2.667, 98.3)
  line L23 (0, 106) -> (-2.667, 106) projected
  line L24 (-11.031, 106) -> (-2.667, 106)
  line L25 (-2.667, 106) -> (-2.667, 113.2675) projected
  line L26 (-2.667, 106) -> (-2.667, 113.2675)
  line L27 (-11.031, 106) -> (-11.031, 113.2675) projected
  line L28 (-2.667, 113.2675) -> (-11.031, 113.2675)
  line L29 (-11.031, 113.2675) -> (-11.031, 106)
  dimension "d134" = 1.3
  dimension "d135" = 6.4
  dimension "d136" = 1.3
  dimension "d137" = 6.4
  constraints: 36 end point, 13 perpendicular, 4 collinear, 2 point on line, 1 vertical
  measures "d134" distance of L0.end L10.end
  measures "d135" distance of L12.end L14.end
  measures "d136" distance of L3.end L18.end
  measures "d137" distance of L19.end L20.end
extrude "Extrusion10" cut sketch "Sketch10" against normal blind 9 contours L6 L5 L4 L2 | L19 L20 L21 L22 | L12 L14 L16 L17
extrude "Extrusion11" cut sketch "Sketch10" against normal blind 156.1 contours L27 L28 L25 L24
sketch "Sketch11" plane through (-9, -9, 0) normal (-1, 0, 0) x (0, 0, 1)
  line L0 (2.667, -89.3) -> (2.667, -95.7) projected
  line L1 (11.031, -89.3) -> (2.667, -89.3) projected
  line L2 (11.031, -95.7) -> (11.031, -89.3) projected
  line L3 (2.667, -95.7) -> (11.031, -95.7) projected
  line L4 (11.031, 7.7) -> (2.667, 7.7) projected
  line L5 (11.031, 1.3) -> (11.031, 7.7) projected
  line L6 (2.667, 1.3) -> (11.031, 1.3) projected
  line L7 (2.667, 7.7) -> (2.667, 1.3) projected
  line L8 (0, 0) -> (13.651, 0) projected
  line L9 (13.651, -88) -> (13.651, 0) projected
  line L10 (13.651, -88) -> (0, -88) projected
  line L11 (0, -88) -> (0, 0) projected
  point P0 (0, 9)
extrude "Extrusion12" cut sketch "Sketch11" against normal blind 9
sketch "Sketch12" plane through (0, 0, 13.651) normal (0, 0, 1) x (1, 0, 0)
  line L0 (129.8502, 0) -> (-9, 0) projected
  line L1 (-9, 0) -> (-9, -9) projected
  line L2 (-9, -9) -> (0, -9) projected
  line L3 (0, -9) -> (0, -97) projected
  line L4 (0, -97) -> (-9, -97) projected
  line L5 (-9, -97) -> (-9, -106) projected
  line L6 (-9, -106) -> (129.8502, -106) projected
  line L7 (129.8502, -106) -> (129.8502, -97) projected
  line L8 (129.8502, -97) -> (120.8502, -97) projected
  line L9 (120.8502, -97) -> (120.8502, -9) projected
  line L10 (120.8502, -9) -> (129.8502, -9) projected
  line L11 (129.8502, -9) -> (129.8502, 0) projected
  circle A0 centre (125.3502, -4.5) radius 1.65 projected
  circle A1 centre (125.3502, -101.5) radius 1.65 projected
  circle A2 centre (-4.5, -101.5) radius 1.65 projected
  circle A3 centre (-4.5, -4.5) radius 1.65 projected
  point P0 (0, 0)
sketch "Sketch13" plane through (0, 0, 1.651) normal (0, 0, 1) x (1, 0, 0)
  circle A0 centre (45.1902, -92.18) radius 3.05 projected
  circle A1 centre (73.6502, -92.18) radius 3.05 projected
  line L0 (41.4402, -98.98) -> (48.9402, -98.98)
  line L1 (48.9402, -98.98) -> (48.9402, -85.38)
  line L2 (48.9402, -85.38) -> (41.4402, -85.38)
  line L3 (41.4402, -85.38) -> (41.4402, -98.98)
  line L4 (41.4402, -98.98) -> (48.9402, -85.38) construction
  line L5 (48.9402, -98.98) -> (41.4402, -85.38) construction
  line L6 (69.9002, -98.98) -> (77.4002, -98.98)
  line L7 (77.4002, -98.98) -> (77.4002, -85.38)
  line L8 (77.4002, -85.38) -> (69.9002, -85.38)
  line L9 (69.9002, -85.38) -> (69.9002, -98.98)
  line L10 (69.9002, -98.98) -> (77.4002, -85.38) construction
  line L11 (77.4002, -98.98) -> (69.9002, -85.38) construction
  line L12 (50.5402, -100.58) -> (39.8402, -100.58)
  line L13 (39.8402, -100.58) -> (39.8402, -83.78)
  line L14 (39.8402, -83.78) -> (50.5402, -83.78)
  line L15 (50.5402, -83.78) -> (50.5402, -100.58)
  line L16 (79.0002, -100.58) -> (68.3002, -100.58)
  line L17 (68.3002, -100.58) -> (68.3002, -83.78)
  line L18 (68.3002, -83.78) -> (79.0002, -83.78)
  line L19 (79.0002, -83.78) -> (79.0002, -100.58)
  point P0 (0, 0)
  dimension "d146" = 7.5
  dimension "d147" = 13.6
  dimension "d148" = 7.5
  dimension "d149" = 1.6
  dimension "d150" = 1.6
  constraints: 40 end point, 8 parallel, 4 midpoint, 4 perpendicular, 2 horizontal, 6 other
  measures "d146" distance of L2.end L1.end
  measures "d147" distance of L1.end L0.end
  measures "d148" distance of L8.end L7.end
  measures "d149" distance between parallel lines of L0 L12
  measures "d150" distance between parallel lines of L6 L16
extrude "Extrusion13" cut sketch "Sketch13" against normal blind 10 contours A0 | A1 | L3 L2 L1 L0 | L9 L8 L7 L6
extrude "Extrusion14" add sketch "Sketch13" along normal blind 9.65 contours A1 | L9 L8 L7 L6 | L16 L17 L18 L19
extrude "Extrusion15" add sketch "Sketch13" along normal blind 9.65 contours A0 | L3 L2 L1 L0 | L12 L13 L14 L15
sketch "Sketch14" plane through (0, 0, 1.651) normal (0, 0, -1) x (-1, 0, 0)
  line L0 (-77.4002, -98.98) -> (-69.9002, -98.98) projected
  line L1 (-69.9002, -98.98) -> (-69.9002, -85.38) projected
  line L2 (-69.9002, -85.38) -> (-77.4002, -85.38) projected
  line L3 (-77.4002, -85.38) -> (-77.4002, -98.98) projected
  line L4 (-48.9402, -98.98) -> (-41.4402, -98.98) projected
  line L5 (-41.4402, -98.98) -> (-41.4402, -85.38) projected
  line L6 (-41.4402, -85.38) -> (-48.9402, -85.38) projected
  line L7 (-48.9402, -85.38) -> (-48.9402, -98.98) projected
  point P0 (0, 0)
extrude "Extrusion16" cut sketch "Sketch14" against normal blind 8
sketch "Sketch15" plane through (0, 0, 9.651) normal (0, 0, -1) x (-1, 0, 0)
  circle A0 centre (-73.6502, -92.18) radius 3.05 projected
  circle A1 centre (-45.1902, -92.18) radius 3.05 projected
  point P0 (0, 0)
extrude "Extrusion17" cut sketch "Sketch15" against normal blind 8
sketch "Sketch16" plane through (0, 0, 13.651) normal (0, 0, 1) x (1, 0, 0)
  line L0 (-48.6937, -126.5536) -> (194.3247, -126.5536)
  line L1 (194.3247, -126.5536) -> (194.3247, 28.5202)
  line L2 (194.3247, 28.5202) -> (-48.6937, 28.5202)
  line L3 (-48.6937, 28.5202) -> (-48.6937, -126.5536)
  point P0 (0, 0)
  constraints: 8 end point, 2 parallel, 1 horizontal, 1 perpendicular
extrude "Extrusion18" cut sketch "Sketch16" against normal blind 5
sketch "Sketch17" plane through (0, 0, 8.651) normal (0, 0, 1) x (1, 0, 0)
  line L0 (50.5402, -100.58) -> (39.8402, -100.58) projected
  line L1 (68.3002, -83.78) -> (79.0002, -83.78) projected
  line L2 (39.8402, -100.58) -> (79.0002, -100.58)
  line L3 (79.0002, -100.58) -> (79.0002, -83.78)
  line L4 (79.0002, -83.78) -> (39.8402, -83.78)
  line L5 (39.8402, -83.78) -> (39.8402, -100.58)
  point P0 (0, 0)
  constraints: 8 end point, 2 parallel, 1 horizontal, 1 perpendicular
extrude "Extrusion19" cut sketch "Sketch17" against normal blind 2.35
sketch "Sketch18" plane through (0, 0, 6.301) normal (0, 0, 1) x (1, 0, 0)
  line L0 (50.5402, -83.78) -> (50.5402, -100.58) projected
  line L1 (39.8402, -100.58) -> (50.5402, -100.58)
  line L2 (50.5402, -100.58) -> (50.5402, -83.78)
  line L3 (50.5402, -83.78) -> (39.8402, -83.78)
  line L4 (39.8402, -83.78) -> (39.8402, -100.58)
  circle A0 centre (45.1902, -92.18) radius 3.05
  line L5 (68.3002, -83.78) -> (79.0002, -83.78) projected
  line L6 (68.3002, -100.58) -> (79.0002, -100.58)
  line L7 (79.0002, -100.58) -> (79.0002, -83.78)
  line L8 (79.0002, -83.78) -> (68.3002, -83.78)
  line L9 (68.3002, -83.78) -> (68.3002, -100.58)
  circle A1 centre (73.6502, -92.18) radius 3.05
  point P0 (0, 0)
  dimension "d165" = 6.1
  constraints: 16 end point, 4 parallel, 2 centre point, 2 horizontal, 2 perpendicular
  measures "d165" diameter of A0
extrude "Extrusion20" add sketch "Sketch18" against normal blind 1.65 contours L0 L1 L4 L3 | A0 | L5 L7 L6 L9 | A1
extrude "Extrusion21" cut sketch "Sketch18" against normal blind 1.65 contours A0 | A1
sketch "Sketch19" plane through (0, 0, 8.651) normal (0, 0, 1) x (1, 0, 0)
  circle A0 centre (-4.5, -4.5) radius 1.65 projected
  line L0 (-9, -7.7) -> (-9, -1.3) projected
  line L1 (-9, -7.7) -> (0, -7.7) projected
  line L2 (0, -7.7) -> (0, -1.3) projected
  line L3 (-9, -1.3) -> (0, -1.3) projected
  circle A1 centre (125.3502, -4.5) radius 1.65 projected
  line L4 (129.8502, -1.3) -> (129.8502, -7.7) projected
  line L5 (129.8502, -1.3) -> (120.8502, -1.3) projected
  line L6 (120.8502, -1.3) -> (120.8502, -7.7) projected
  line L7 (129.8502, -7.7) -> (120.8502, -7.7) projected
  circle A2 centre (125.3502, -101.5) radius 1.65 projected
  line L8 (129.8502, -98.3) -> (129.8502, -104.7) projected
  line L9 (129.8502, -98.3) -> (120.8502, -98.3) projected
  line L10 (120.8502, -98.3) -> (120.8502, -104.7) projected
  line L11 (129.8502, -104.7) -> (120.8502, -104.7) projected
  circle A3 centre (-4.5, -101.5) radius 1.65 projected
  line L12 (-9, -104.7) -> (-9, -98.3) projected
  line L13 (-9, -104.7) -> (0, -104.7) projected
  line L14 (0, -104.7) -> (0, -98.3) projected
  line L15 (-9, -98.3) -> (0, -98.3) projected
  point P0 (0, 0)
extrude "Extrusion22" add sketch "Sketch19" against normal blind 1.9 contours L0 L3 L2 L1 | L4 L7 L6 L5 | A2 | L8 L11 L10 L9 | L12 L15 L14 L13
sketch "Sketch20" plane through (0, 0, 8.651) normal (0, 0, 1) x (1, 0, 0)
  circle A0 centre (125.3502, -101.5) radius 1.65 projected
  point P0 (0, 0)
extrude "Extrusion23" cut sketch "Sketch20" against normal blind 17.775
sketch "Sketch21" plane through (129.8502, -106, 0) normal (1, 0, 0) x (0, 0, -1)
  line L0 (-8.651, 106) -> (0, 106) projected
  line L1 (0, 97) -> (0, 106) projected
  line L2 (-8.651, 9) -> (0, 9) projected
  line L3 (0, 6.15) -> (0, 2.85) projected
  line L4 (-6.751, 7.7) -> (-6.751, 1.3) projected
  line L5 (-2.667, 1.3) -> (-6.751, 1.3) projected
  line L6 (-2.667, 7.7) -> (-2.667, 1.3) projected
  line L7 (-6.751, 7.7) -> (-2.667, 7.7) projected
  line L8 (-6.751, 104.7) -> (-6.751, 98.3) projected
  line L9 (-2.667, 98.3) -> (-6.751, 98.3) projected
  line L10 (-2.667, 104.7) -> (-2.667, 98.3) projected
  line L11 (-6.751, 104.7) -> (-2.667, 104.7) projected
  line L12 (-6.9505, 98.3) -> (-1.7005, 98.3)
  line L13 (-1.7005, 98.3) -> (-1.7005, 104.7)
  line L14 (-1.7005, 104.7) -> (-6.9505, 104.7)
  line L15 (-6.9505, 104.7) -> (-6.9505, 98.3)
  line L16 (-6.9505, 98.3) -> (-1.7005, 104.7) construction
  line L17 (-1.7005, 98.3) -> (-6.9505, 104.7) construction
  line L18 (-6.9505, 1.3) -> (-1.7005, 1.3)
  line L19 (-1.7005, 1.3) -> (-1.7005, 7.7)
  line L20 (-1.7005, 7.7) -> (-6.9505, 7.7)
  line L21 (-6.9505, 7.7) -> (-6.9505, 1.3)
  line L22 (-6.9505, 1.3) -> (-1.7005, 7.7) construction
  line L23 (-1.7005, 1.3) -> (-6.9505, 7.7) construction
  point P0 (-4.3255, 106)
  point P1 (0, 101.5)
  point P2 (-4.3255, 9)
  point P3 (0, 4.5)
  point P4 (-4.3255, 101.5)
  point P5 (-4.3255, 4.5)
  dimension "d174" = 5.25
  constraints: 24 end point, 8 midpoint, 4 parallel, 2 horizontal, 2 perpendicular, 1 point on line
  measures "d174" distance of L14.end L13.end
extrude "Extrusion24" cut sketch "Sketch21" against normal blind 9
sketch "Sketch23" plane through (0, 0, 0) normal (0, 0, -1) x (-1, 0, 0)
  line L0 (9, 0) -> (-129.8502, 0) projected
  line L1 (-120.8502, 0) -> (0, 0)
  line L2 (9, -106) -> (-129.8502, -106) projected
  line L3 (0, -106) -> (-120.8502, -106)
  line L4 (-118.8502, -2) -> (-2, -2)
  line L5 (-2, -2) -> (-2, -104)
  line L6 (-2, -104) -> (-118.8502, -104)
  line L7 (-118.8502, -104) -> (-118.8502, -2)
  line L8 (-129.8502, -97) -> (-120.8502, -97) projected
  line L9 (-129.8502, -106) -> (-129.8502, -97) projected
  line L10 (9, -97) -> (9, -106) projected
  line L11 (0, -97) -> (9, -97) projected
  line L12 (9, -9) -> (0, -9) projected
  line L13 (9, 0) -> (9, -9) projected
  line L14 (-129.8502, -9) -> (-129.8502, 0) projected
  line L15 (-120.8502, -9) -> (-129.8502, -9) projected
  circle A0 centre (-125.3502, -4.5) radius 1.65 projected
  circle A1 centre (4.5, -4.5) radius 1.65 projected
  circle A2 centre (4.5, -101.5) radius 1.65 projected
  circle A3 centre (-125.3502, -101.5) radius 1.65 projected
  line L16 (0, -9) -> (9, -9) projected
  line L17 (-129.8502, -9) -> (-120.8502, -9) projected
  line L18 (-120.8502, -9) -> (-120.8502, -97)
  line L19 (0, -97) -> (0, -9)
  constraints: 16 end point, 2 perpendicular, 2 point on line, 1 collinear, 1 horizontal, 1 parallel, 1 vertical
extrude "Extrusion26" add sketch "Sketch23" along normal blind 1.39
sketch "Sketch24" plane through (129.8502, -106, 8.651) normal (1, 0, 0) x (0, 0, -1)
  line L0 (0, 106) -> (10.041, 106) projected
  line L1 (1.7005, 98.3) -> (1.7005, 104.7) projected
  line L2 (0, 106) -> (0, 97) projected
  line L3 (8.2995, 98.3) -> (1.7005, 98.3)
  line L4 (1.7005, 98.3) -> (1.7005, 104.7)
  line L5 (1.7005, 104.7) -> (8.2995, 104.7)
  line L6 (8.2995, 104.7) -> (8.2995, 98.3)
  line L7 (5, 104.4404) -> (5, 87.26) projected
  line L8 (8.2995, 98.3) -> (1.7005, 104.7) construction
  line L9 (1.7005, 98.3) -> (8.2995, 104.7) construction
  line L10 (10.041, 0) -> (0, 0) projected
  line L11 (1.7005, 1.3) -> (1.7005, 7.7) projected
  line L12 (8.2995, 7.7) -> (1.7005, 7.7)
  line L13 (1.7005, 7.7) -> (1.7005, 1.3)
  line L14 (1.7005, 1.3) -> (8.2995, 1.3)
  line L15 (8.2995, 1.3) -> (8.2995, 7.7)
  line L16 (5, 2.8371) -> (5, 26.25) projected
  line L17 (8.2995, 7.7) -> (1.7005, 1.3) construction
  line L18 (1.7005, 7.7) -> (8.2995, 1.3) construction
  point P0 (8.651, 106)
  point P1 (5.0205, 106)
  point P2 (1.7005, 101.5)
  point P3 (5, 101.5)
  point P4 (5.0205, 0)
  point P5 (1.7005, 4.5)
  point P6 (5, 4.5)
  dimension "d182" = 1.7005
  constraints: 24 end point, 8 midpoint, 4 parallel, 2 horizontal, 2 perpendicular, 2 point on line
  measures "d182" distance between parallel lines of L2 L1
extrude "Extrusion27" cut sketch "Sketch24" against normal blind 9